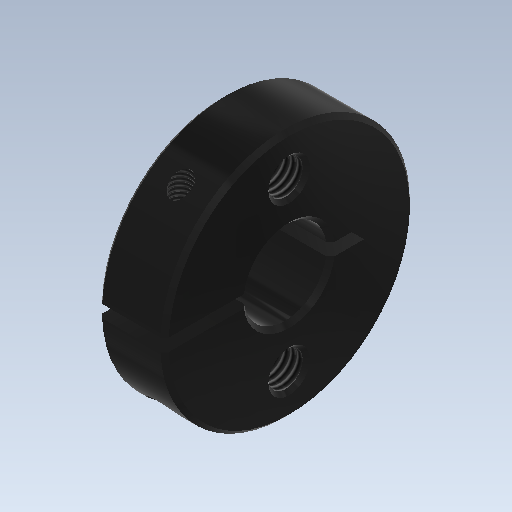
# Autodesk Inventor part: SSCSW10-8b
Saved by Autodesk Inventor 2021 (Build 250183000, 183)
## iProperties
Category: PARTsolutions
Company: MISUMI
Part Number: SSCSW10-8b
Material: 鉄、鋳鉄
Catalog Web Link: www.cadenas.de
Description: SCSW, PSCSW, SSCSW-b-Shaft Collars - 2 Holes/2 Taps - 2-Tapped (Coarse Thread)
Vendor: MISUMI
Document SubType Name: Modeling
Designer: partserver
Manufacturer: MISUMI
Mass: 30.9021 g
Surface Area: 27.1004 cm^2
Volume: 4.32197 cm^3
Density: 7.15 g/cm^3
Appearance: 鉄 灰色
PSOL_IDENT_0: {$CADENAS_DATA\23d-libs\misumi\metric\03_set_collars\scsw_b.prj},185 {VTYP=3D},{NB=SSCSW10-8b},{LINA=
PSOL_IDENT_1: SSCSW10-8b},{NN=SCSW, PSCSW, SSCSW-b},{DATE=30.03.2018 01:14:49},{GEOMDATE=24.02.2016 04:36:42},{VER
PSOL_IDENT_2: SION=},{LINEID=60},{WBVAR=MAT,ST,BS},{WBNUMERIC=BS}  {NB=SSCSW10-8b},{LINA=SSCSW10-8b},{KT=DUMMY},{P
PSOL_IDENT_3: N=SSCSW10-8},{TYPE=SSCSW},{MAT=304},{ST=-},{AC=Hexagon Socket Head Set Screw 1 Pc. (304 Stainless St
PSOL_IDENT_4: eel) },{D=10},{BS=8},{D1=30},{M=M3},{THMD=3},{THDMIN=2.459},{ST0='-','-'},{B1=8,10,12},{DD=3.4},{R=3
PSOL_IDENT_5: .00},{W=1.5},{X=9.0},{Y=5.0},{Z=8~10},{S=5.5},{P=20},{C=0.5},{L=10},{M1=M5},{ZZ=9},{THMD1=5},{THDMIN
PSOL_IDENT_6: 1=4.134}
NB: SSCSW10-8b
NN: SCSW, PSCSW, SSCSW-b
NT: Shaft Collars - 2 Holes/2 Taps - 2-Tapped (Coarse Thread)
NBSYN: $PN.b
LINA: SSCSW10-8b
CATALOG: Misumi
PN: SSCSW10-8
MAT: SUS304 Equivalent
ST: -
AC: Hexagon Socket Head Set Screw 1 Pc. (304 Stainless Steel)
D: 10
BS: 8
D1: 30
M: M3
DD: 3.4
R: 3
W: 1.5
X: 9
Y: 5
Z: 8~10
S: 5.5
P: 20
M1: M5
SUPPLIER: MISUMI
ARTICLENO: SSCSW10-8b
BOMINFO: SSCSW10-8b
CREATOR: CADENAS GmbH
d13: 0.000 mm
Title: SSCSW10-8b
Author: Cadenas PARTsolutions
Comments: Shaft Collars - 2 Holes/2 Taps - 2-Tapped (Coarse Thread)
Autodesk Inventor part; units mm, degrees
sketch "Sketch_1" plane through (0, 0, 0) normal (0, 0, 1) x (1, 0, 0)
  line L0 (4, 0) -> (-4, 0)
  line L1 (-4, 14.5) -> (-4, 5.5)
  line L2 (-4, 5.5) -> (-3.5, 5)
  line L3 (-3.5, 5) -> (3.5, 5)
  line L4 (3.5, 5) -> (4, 5.5)
  line L5 (4, 5.5) -> (4, 14.5)
  line L6 (4, 14.5) -> (3.5, 15)
  line L7 (3.5, 15) -> (-3.5, 15)
  line L8 (-3.5, 15) -> (-4, 14.5)
  constraints: 18 end point
revolve "Revolution1" add sketch "Sketch_1" angle 360 about axis through (4, 0, 0) along (1, 0, 0)
sketch "Sketch_2" plane through (0, 0, 0) normal (1, 0, 0) x (0, 1, 0)
  line L0 (-15, 0.75) -> (-15, -0.75)
  line L1 (-15, -0.75) -> (9, -0.75)
  line L2 (9, -0.75) -> (9, 0.75)
  line L3 (9, 0.75) -> (-15, 0.75)
  constraints: 8 end point
extrude "Extrusion1" cut sketch "Sketch_2" along normal mid plane 8
sketch "Sketch_3" plane through (0, 0, 0) normal (1, 0, 0) x (0, 1, 0)
  line L0 (-9, 15) -> (-9, 0)
  line L1 (-9, 0) -> (-10.7, 0)
  line L2 (-10.7, 0) -> (-10.7, 5)
  line L3 (-10.7, 5) -> (-12, 5)
  line L4 (-12, 5) -> (-12, 15)
  line L5 (-12, 15) -> (-9, 15)
  line L6 (-9, 15) -> (-9, 0)
  constraints: 14 end point
revolve "Revolution2" cut sketch "Sketch_3" angle 360 about axis through (0, -9, 15) along (0, 0, 1)
sketch "Sketch_4" plane through (0, 0, 0) normal (1, 0, 0) x (0, 1, 0)
  line L0 (-9, -14.25) -> (-9, -0.75)
  line L1 (-9, -0.75) -> (-7.5, -0.75)
  line L2 (-7.5, -0.75) -> (-7.7705, -1.0205)
  line L3 (-7.7705, -1.0205) -> (-7.7705, -14.25)
  line L4 (-7.7705, -14.25) -> (-9, -14.25)
  line L5 (-9, -14.25) -> (-9, -0.75)
  constraints: 12 end point
revolve "Revolution3" cut sketch "Sketch_4" angle 360 about axis through (0, -9, -14.25) along (0, 0, -1)
thread "Thread1" size "M3x0.5" class "6H" standard "ISO Metric profile" length 11.9699
sketch "Sketch_7" plane through (0, 0, -10) normal (0, 0, 1) x (1, 0, 0)
  line L0 (4, 0) -> (-4, 0)
  line L1 (-4, 0) -> (-4, 2.5)
  line L2 (-4, 2.5) -> (-3.567, 2.067)
  line L3 (-3.567, 2.067) -> (3.567, 2.067)
  line L4 (3.567, 2.067) -> (4, 2.5)
  line L5 (4, 2.5) -> (4, 0)
  line L6 (4, 0) -> (-4, 0)
  constraints: 14 end point
revolve "Revolution4" cut sketch "Sketch_7" angle 360 about axis through (4, 0, -10) along (1, 0, 0)
thread "Thread2" size "M5x0.8" class "6H" standard "ISO Metric profile" full length
sketch "Sketch_8" plane through (0, 0, 10) normal (0, 0, 1) x (1, 0, 0)
  line L0 (4, 0) -> (-4, 0)
  line L1 (-4, 0) -> (-4, 2.5)
  line L2 (-4, 2.5) -> (-3.567, 2.067)
  line L3 (-3.567, 2.067) -> (3.567, 2.067)
  line L4 (3.567, 2.067) -> (4, 2.5)
  line L5 (4, 2.5) -> (4, 0)
  line L6 (4, 0) -> (-4, 0)
  constraints: 14 end point
revolve "Revolution5" cut sketch "Sketch_8" angle 360 about axis through (4, 0, 10) along (1, 0, 0)
thread "Thread3" size "M5x0.8" class "6H" standard "ISO Metric profile" full length
ref_plane "body_screw_XY" through (0, -9, 5) normal (0, 0, 1) x (1, 0, 0)
ref_plane "body_screw_YZ" through (0, -9, 5) normal (1, 0, 0) x (0, 1, 0)
ref_plane "body_screw_ZX" through (0, -9, 5) normal (0, 1, 0) x (0, 0, 1)
body "Solid1"
